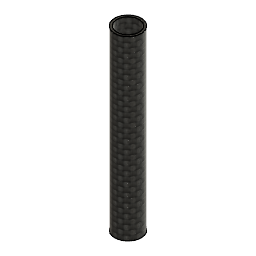
axial_generator (Autodesk Fusion 360 archive; units mm, degrees)
design "carbon_fibre_armature"
Autodesk Fusion 360 part; units mm, degrees
sketch "Sketch1" plane through (0, 0, 0) normal (0, 1, 0) x (1, 0, 0)
  circle A0 centre (0, 0) radius 5
  circle A1 centre (0, 0) radius 6
  dimension "d1" = 10
  dimension "d2" = 12
  constraint coincident A0.centre A1.centre
  measures "d1" diameter of A0
  measures "d2" diameter of A1
extrude "Extrude1" add sketch "Sketch1" along normal blind 80

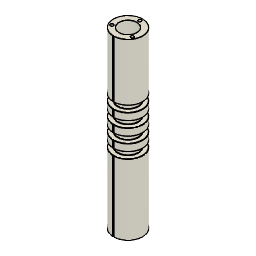
design "stator"
Autodesk Fusion 360 part; units mm, degrees
sketch "cross_sectional" plane through (0, 0, 0) normal (1, 0, 0) x (0, 0, -1)
  line L0 (0, 0) -> (-6.6, 0) construction
  line L1 (-6.6, 0) -> (-7.6, 0)
  line L2 (-6.6, 0) -> (-6.6, 140)
  line L3 (-7.6, 0) -> (-11, 0)
  line L4 (-11, 0) -> (-11, 140)
  line L5 (-11, 140) -> (-6.6, 140)
  dimension "d1" = 6.6
  dimension "d2" = 1
  dimension "d3" = 140
  dimension "d4" = 3.4
  constraint coincident L0.start origin
  constraint horizontal L0
  constraint parallel L0 L1
  constraint perpendicular L0 L2
  constraint perpendicular L2 L3
  constraint perpendicular L3 L4
  constraint perpendicular L2 L5
  measures "d1" distance of L0.start L0.end
  measures "d2" distance of L0.end L1.end
  measures "d3" distance of L0.end L2.end
  measures "d4" distance of L1.end L3.end
revolve "Revolve1" add sketch "cross_sectional" angle 360 about axis through (0, 1.75, 0) along (0, 1, 0)
ref_plane "WorkPlane1" through (0, 52.7, 0) normal (0, 1, 0) x (0, 0, 1)
sketch "outer_coils" plane through (0, 52.7, 0) normal (0, 1, 0) x (1, 0, 0)
  circle A0 centre (0, 0) radius 7.6
  circle A1 centre (0, 0) radius 11
  dimension "d7" = 15.2
  constraint coincident A0.centre A1.centre
  measures "d7" diameter of A0
extrude "Extrude1" cut sketch "outer_coils" along normal blind 4.6
fillet "Fillet1" radius 0.2 4 edges at (-7.0857, 52.7, -2.7483) (3.9778, 52.7, -10.2556) (-7.0857, 57.3, -2.7483) (-3.9778, 57.3, -10.2556)
pattern_linear "R-Pattern1" count 4 spacing 10 along (0, 1, 0) of 7 faces at (0.7309, 52.7, 9.7525) (-9.2394, 52.5209, 5.9674) (7.1547, 52.8269, 2.6041) (7.5622, 54.3, 0.7567) (7.1547, 57.1731, 2.6041) (-0.7309, 57.3, 9.7525) (-10.9135, 57.4791, -1.3676)
ref_plane "WorkPlane2" through (0, 5, 0) normal (0, -1, 0) x (0, 0, -1)
sketch "inter_dia" plane through (0, 5, 0) normal (0, -1, 0) x (-1, 0, 0)
  circle A0 centre (0, 0) radius 6.6
  dimension "d17" = 13.2
  constraint coincident A0.centre origin
  measures "d17" diameter of A0
extrude "Extrude2" add sketch "inter_dia" against normal blind 5
sketch "magnet_dia" plane through (0, 5, 0) normal (0, -1, 0) x (1, 0, 0)
  circle A0 centre (0, 0) radius 6.25
  circle A1 centre (0, 0) radius 6.6
  dimension "d20" = 12.5
  measures "d20" diameter of A0
sketch "Sketch8" plane through (0, 0, 0) normal (0, -1, 0) x (1, 0, 0)
  circle A0 centre (0, 0) radius 6.6
  circle A1 centre (0, 0) radius 11
  circle A2 centre (0, 0) radius 6
  circle A3 centre (0, 0) radius 6.6
  dimension "d43" = 12
  constraint coincident A0.centre A1.centre
  constraint concentric A2 A3
  measures "d43" diameter of A2
extrude "Extrude8" add sketch "Sketch8" against normal blind 5 contours A0 A3
extrude "Extrude3" add sketch "magnet_dia" along normal blind 5
fillet "Fillet2" radius 0.2 1 edges at (-10.2556, 0, 3.9778)
fillet "Fillet2" radius 0.2 1 edges at (2.3867, 10, -6.1534)
sketch "wire_dia" plane through (0, 52.7, 0) normal (0, 1, 0) x (-1, 0, 0)
  circle A0 centre (0, 0) radius 7.8
  circle A1 centre (0, 0) radius 10.8
  circle A2 centre (0, 0) radius 11
  circle A3 centre (0, 11) radius 0.4
  dimension "d27" = 0.8
  constraint concentric A0 A2
  constraint coincident A2 A3.centre
  measures "d27" diameter of A3
extrude "Extrude4" cut sketch "wire_dia" along normal blind 87.3 contours A1 A3 | A1 A2 A3 | A2 A3 picked at (0, 10.7329) picked at (0.0381, 10.9326)
extrude "Extrude5" cut sketch "wire_dia" against normal blind 62.5 contours A1 A3 | A1 A2 A3 | A2 A3 picked at (0, 10.7329) picked at (0.0381, 10.9326)
fillet "Fillet3" radius 0.1 37 edges at (0, 52.7, 10.6) (0.3941, 52.6443, 10.9314) (0.3999, 26.35, 10.9927) (0.3941, 0.0557, 10.9314) (0, 0, 10.6) (-0.3941, 0.0557, 10.9314) (-0.3999, 26.35, 10.9927) (-0.3941, 52.6443, 10.9314) (0, 62.7, 10.6) (0.3941, 62.6443, 10.9314) (0.3999, 60, 10.9927) (0.3941, 57.3557, 10.9314) (0, 57.3, 10.6) (-0.3941, 57.3557, 10.9314) (-0.3999, 60, 10.9927) (-0.3941, 62.6443, 10.9314) (0.3941, 72.6443, 10.9314) (0.3999, 70, 10.9927) (0.3941, 67.3557, 10.9314) (0, 67.3, 10.6) (-0.3941, 67.3557, 10.9314) (-0.3999, 70, 10.9927) (-0.3941, 72.6443, 10.9314) (0, 72.7, 10.6) (0.3941, 82.6443, 10.9314) (0.3999, 80, 10.9927) (0.3941, 77.3557, 10.9314) (0, 77.3, 10.6) (-0.3941, 77.3557, 10.9314) (-0.3999, 80, 10.9927) (-0.3941, 82.6443, 10.9314) (0, 82.7, 10.6) (0.3999, 113.75, 10.9927) (0.3941, 87.3557, 10.9314) (0, 87.3, 10.6) (-0.3941, 87.3557, 10.9314) (-0.3999, 113.75, 10.9927)
sketch "Sketch6" plane through (0, 140, 0) normal (0, 1, 0) x (-1, 0, 0)
  circle A0 centre (0, 0) radius 6.6
  arc A1 (0.492, 10.989) -> (0.39, 10.9113) centre (0.4875, 10.8891) ccw
  arc A2 (-0.39, 10.9113) -> (0.39, 10.9113) centre (0, 11) ccw
  arc A3 (-0.39, 10.9113) -> (-0.492, 10.989) centre (-0.4875, 10.8891) ccw
  arc A4 (-0.492, 10.989) -> (0.492, 10.989) centre (0, 0) ccw
  circle A5 centre (0, 0) radius 6.6
  circle A6 centre (0, 0) radius 11
  circle A7 centre (0, 0) radius 9
  constraint concentric A0 A5
  constraint concentric A5 A6
  constraint concentric A5 A7
extrude "Extrude6" cut sketch "Sketch6" against normal blind 10 contours A1 A2 A3 A4 A6 | A7
sketch "Sketch7" plane through (0, 130, 0) normal (0, 1, 0) x (-1, 0, 0)
  circle A0 centre (0, 0) radius 6.6
  arc A1 (-0.39, 10.9113) -> (-0.492, 10.989) centre (-0.4875, 10.8891) ccw
  arc A2 (-0.492, 10.989) -> (0.492, 10.989) centre (0, 0) ccw
  arc A3 (0.492, 10.989) -> (0.39, 10.9113) centre (0.4875, 10.8891) ccw
  arc A4 (-0.39, 10.9113) -> (0.39, 10.9113) centre (0, 11) ccw
  circle A5 centre (0, 0) radius 8.8
  circle A6 centre (0, -8.8) radius 1.05
  circle A7 centre (7.621, 4.4) radius 1.05
  circle A8 centre (-7.621, 4.4) radius 1.05
  dimension "d36" = 17.6
  dimension "d37" = 2.1
  dimension "d39" = 360
  constraint coincident A0.centre A2.centre
  constraint coincident A5 A6.centre
  measures "d36" diameter of A5
  measures "d37" diameter of A6
extrude "Extrude7" cut sketch "Sketch7" against normal blind 10 contours A5 A7 | A5 A7 | A5 A6 | A5 A6 | A5 A8 | A5 A8
chamfer "Chamfer1" distance 0.1 angle 45 11 edges at (-6.6421, 130, 4.7797) (-2.3867, 130, -6.1534) (0, 130, -11) (0.4269, 130, 10.9686) (0, 130, 10.6) (-0.4269, 130, 10.9686) (0.9789, 130, -8.4203) (8.6, 130, 4.7797) (0.9789, 120, -8.4203) (-6.6421, 120, 4.7797) (8.6, 120, 4.7797)
fillet "Fillet4" radius 0.2 1 edges at (-5.594, 0, 2.1697)
sketch "Sketch9" plane through (0, 0, 0) normal (0, 1, 0) x (1, 0, 0)
  circle A0 centre (0, 0) radius 40
  circle A1 centre (0, 0) radius 10.8167
  dimension "d48" = 80
  constraint coincident A0.centre A1.centre
  constraint concentric A0 A1
  measures "d48" diameter of A0
equation "d1 = 13.2 mm / 2"
equation "d3 = 80 mm + 60 mm"
equation "d6 = 30.00 mm + 20 mm + 2.7 mm"
equation "d7 = ( ( 6.6 + 1 ) * 2 ) * 1 mm"
equation "d36 = ( ( 22.000 + 13.2 ) / 2 ) * 1 mm"

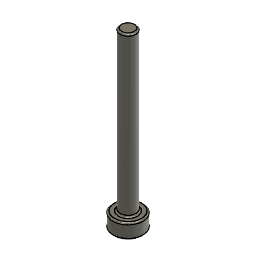
design "m2 by 20mm bolt"
Autodesk Fusion 360 part; units mm, degrees
sketch "Sketch1" plane through (0, 0, 0) normal (0, 1, 0) x (1, 0, 0)
  circle A0 centre (0, 0) radius 1.9
  line L0 (0, 1.5) -> (-1.299, 0.75)
  line L1 (-1.299, 0.75) -> (-1.299, -0.75)
  line L2 (-1.299, -0.75) -> (0, -1.5)
  line L3 (0, -1.5) -> (1.299, -0.75)
  line L4 (1.299, -0.75) -> (1.299, 0.75)
  line L5 (1.299, 0.75) -> (0, 1.5)
  circle A1 centre (0, 0) radius 1
  dimension "d1" = 3.8
  dimension "d2" = 1.5
  dimension "d3" = 2
  constraint coincident A0.centre A1.centre
  measures "d1" diameter of A0
  measures "d2" distance of L0.start A0.centre
  measures "d3" diameter of A1
extrude "Extrude1" add sketch "Sketch1" along normal blind 20 contours A0 | L0 L1 L2 L3 L4 L5 | A1 makes body 1
extrude "Extrude2" cut sketch "Sketch1" along normal blind 20 contours A0 | L0 L1 L2 L3 L4 L5 bodies 1
extrude "Extrude3" add sketch "Sketch1" against normal blind 1.9 separate body contours A0 | L0 L1 L2 L3 L4 L5 makes body 2
extrude "Extrude4" cut sketch "Sketch1" against normal blind 1.9 contours L0 L1 L2 L3 L4 L5 | A1 bodies 2
extrude "Extrude5" add sketch "Sketch1" against normal blind 1 contours L0 L1 L2 L3 L4 L5 | A1 bodies 1 2
chamfer "Chamfer1" distance 0.1 angle 45 12 edges at (0.6495, -1.9, 1.125) (-0.6495, -1.9, -1.125) (0.6495, -1.9, -1.125) (0.6495, -1, -1.125) (-0.6495, -1, -1.125) (0.6495, -1, 1.125) (-0.6495, -1.9, 1.125) (-0.6495, -1, 1.125) (-1.299, -1, 0) (-1.299, -1.9, 0) (1.299, -1, 0) (1.299, -1.9, 0) on bodies 1 2
fillet "Fillet1" radius 0.2 4 edges at (-1.7714, 0, 0.6871) (-1.7714, -1.9, -0.6871) (-0.9323, 20, 0.3616) (-0.9323, 0, -0.3616) on bodies 1 2

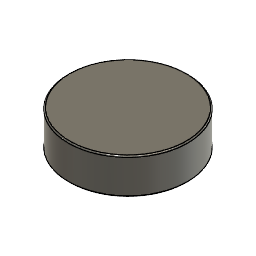
design "10mm by 3mm magnet"
Autodesk Fusion 360 part; units mm, degrees
sketch "Sketch1" plane through (0, 0, 0) normal (0, 1, 0) x (1, 0, 0)
  circle A0 centre (0, 0) radius 5
  dimension "d1" = 10
  constraint coincident A0.centre origin
  measures "d1" diameter of A0
extrude "Extrude1" add sketch "Sketch1" along normal blind 3
fillet "Fillet1" radius 0.1 2 edges at (-4.6616, 3, 1.8081) (-4.6616, 0, 1.8081)

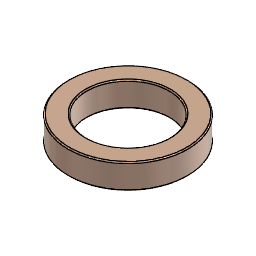
design "coil"
Autodesk Fusion 360 part; units mm, degrees
sketch "Sketch1" plane through (0, 0, 0) normal (0, 1, 0) x (1, 0, 0)
  circle A0 centre (0, 0) radius 11
  circle A1 centre (0, 0) radius 7.6
  dimension "d1" = 22
  dimension "d2" = 15.2
  constraint coincident A0.centre A1.centre
  constraint concentric A0 A1
  measures "d1" diameter of A0
  measures "d2" diameter of A1
extrude "Extrude1" add sketch "Sketch1" along normal blind 4.6
fillet "Fillet1" radius 0.2 4 edges at (-7.0857, 4.6, -2.7483) (-7.0857, 0, -2.7483) (-10.2556, 0, 3.9778) (-10.2556, 4.6, 3.9778)
equation "d1 = ( 11 * 2 ) * 1 mm"

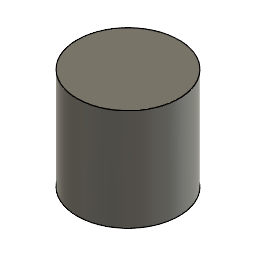
design "10mm by 10mm magnets"
Autodesk Fusion 360 part; units mm, degrees
sketch "Sketch1" plane through (0, 0, 0) normal (0, 1, 0) x (1, 0, 0)
  circle A0 centre (0, 0) radius 5
  dimension "d1" = 10
  constraint coincident A0.centre origin
  measures "d1" diameter of A0
extrude "Extrude1" add sketch "Sketch1" along normal blind 10

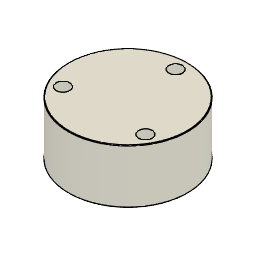
design "stator_end_cap"
Autodesk Fusion 360 part; units mm, degrees
sketch "Sketch1" plane through (0, 0, 0) normal (0, 1, 0) x (1, 0, 0)
  circle A0 centre (0, 0) radius 11
  circle A1 centre (0, 0) radius 8.8
  circle A2 centre (0, 8.8) radius 1.25
  circle A3 centre (-7.621, -4.4) radius 1.25
  circle A4 centre (7.621, -4.4) radius 1.25
  circle A5 centre (0, 0) radius 6
  dimension "d1" = 22
  dimension "d2" = 17.6
  dimension "d3" = 2.5
  dimension "d5" = 360
  dimension "d6" = 12
  constraint coincident A0.centre A1.centre
  constraint concentric A0 A1
  constraint coincident A1 A2.centre
  constraint concentric A1 A5
  measures "d1" diameter of A0
  measures "d2" diameter of A1
  measures "d3" diameter of A2
  measures "d6" diameter of A5
extrude "Extrude1" add sketch "Sketch1" along normal blind 10 contours A0 | A1 A2 A3 A4 | A1 A2 | A1 A2 | A1 A4 | A1 A4 | A1 A3 | A1 A3 | A5
extrude "Extrude2" cut sketch "Sketch1" along normal blind 10 contours A1 A2 | A1 A2 | A1 A4 | A1 A4 | A1 A3 | A1 A3
extrude "Extrude3" cut sketch "Sketch1" along normal blind 5 contours A5
fillet "Fillet1" radius 0.1 6 edges at (-10.2556, 0, 3.9778) (6.4556, 0, 4.852) (-1.1654, 0, -8.348) (-8.7864, 0, 4.852) (-5.594, 0, 2.1697) (-10.2556, 10, 3.9778)
equation "d1 = ( 11 * 2 ) * 1 mm"
